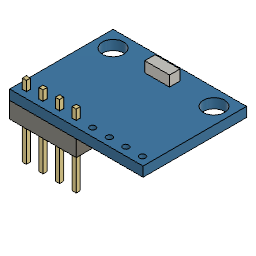
Case_Gyro_Sensor (Autodesk Fusion 360 archive; units mm, degrees)
design "GY-521_MPU6050"
description: Open CASCADE Model
Autodesk Fusion 360 part; units mm, degrees
sketch "Sketch1" plane through (0, 0, 0) normal (0, 0, 1) x (1, 0, 0)
  line L0 (-9.21, -6.355) -> (-8.57, -6.355)
  line L1 (-8.57, -6.355) -> (-8.57, -6.995)
  line L2 (-8.57, -6.995) -> (-9.21, -6.995)
  line L3 (-9.21, -6.995) -> (-9.21, -6.355)
  circle A0 centre (-7.725, 5.425) radius 1.625
  circle A1 centre (7.725, 5.425) radius 1.625
  line L4 (-10.225, 7.925) -> (10.225, 7.925)
  line L5 (10.225, 7.925) -> (10.225, -7.925)
  line L6 (10.225, -7.925) -> (-10.225, -7.925)
  line L7 (-10.225, -7.925) -> (-10.225, 7.925)
  line L8 (-6.03, -6.995) -> (-6.67, -6.995)
  line L9 (-6.67, -6.995) -> (-6.67, -6.355)
  line L10 (-6.67, -6.355) -> (-6.03, -6.355)
  line L11 (-6.03, -6.355) -> (-6.03, -6.995)
  line L12 (-3.49, -6.995) -> (-4.13, -6.995)
  line L13 (-4.13, -6.995) -> (-4.13, -6.355)
  line L14 (-4.13, -6.355) -> (-3.49, -6.355)
  line L15 (-3.49, -6.355) -> (-3.49, -6.995)
  line L16 (-0.95, -6.995) -> (-1.59, -6.995)
  line L17 (-1.59, -6.995) -> (-1.59, -6.355)
  line L18 (-1.59, -6.355) -> (-0.95, -6.355)
  line L19 (-0.95, -6.355) -> (-0.95, -6.995)
  line L20 (1.59, -6.995) -> (0.95, -6.995) construction
  line L21 (0.95, -6.995) -> (0.95, -6.355) construction
  line L22 (0.95, -6.355) -> (1.59, -6.355) construction
  line L23 (1.59, -6.355) -> (1.59, -6.995) construction
  line L24 (4.13, -6.995) -> (3.49, -6.995) construction
  line L25 (3.49, -6.995) -> (3.49, -6.355) construction
  line L26 (3.49, -6.355) -> (4.13, -6.355) construction
  line L27 (4.13, -6.355) -> (4.13, -6.995) construction
  line L28 (6.67, -6.995) -> (6.03, -6.995) construction
  line L29 (6.03, -6.995) -> (6.03, -6.355) construction
  line L30 (6.03, -6.355) -> (6.67, -6.355) construction
  line L31 (6.67, -6.355) -> (6.67, -6.995) construction
  line L32 (9.21, -6.995) -> (8.57, -6.995) construction
  line L33 (8.57, -6.995) -> (8.57, -6.355) construction
  line L34 (8.57, -6.355) -> (9.21, -6.355) construction
  line L35 (9.21, -6.355) -> (9.21, -6.995) construction
  line L36 (-0.95, -6.675) -> (0.95, -6.675) construction
  line L37 (-10.225, -5.425) -> (10.225, -5.425)
  line L38 (10.225, -5.425) -> (10.225, -7.925)
  line L39 (10.225, -7.925) -> (-10.225, -7.925)
  line L40 (-10.225, -7.925) -> (-10.225, -5.425)
  line L41 (0, -5.425) -> (0, -7.925)
  circle A2 centre (1.27, -6.675) radius 0.4525
  circle A3 centre (3.81, -6.675) radius 0.4525
  circle A4 centre (6.35, -6.675) radius 0.4525
  circle A5 centre (8.89, -6.675) radius 0.4525
  line L42 (-2.025, 6.175) -> (1.775, 6.175)
  line L43 (1.775, 6.175) -> (1.775, 4.575)
  line L44 (1.775, 4.575) -> (-2.025, 4.575)
  line L45 (-2.025, 4.575) -> (-2.025, 6.175)
  point P0 (0, -6.675)
  point P1 (0, -5.425)
  point P2 (10.225, 0)
  point P3 (9.21, -6.675)
  point P4 (10.225, -6.675)
  dimension "d1" = 0.64
  dimension "d4" = 2.54
  dimension "d5" = 0
  dimension "d7" = 2.5
  dimension "d8" = 3.25
  dimension "d9" = 2.5
  dimension "d10" = 2.5
  dimension "d11" = 2.5
  dimension "d12" = 15.85
  dimension "d21" = 12
  dimension "d22" = 12.25
  dimension "d23" = 1.6
  dimension "d24" = 1.75
  dimension "d27" = 20.45
  constraint horizontal L0
  constraint vertical L1
  constraint horizontal L2
  constraint vertical L3
  constraint equal L0 L1
  constraint horizontal L4
  constraint vertical L5
  constraint horizontal L6
  constraint vertical L7
  constraint equal A0 A1
  constraint horizontal A0.centre A1.centre
  constraint midpoint L19 L36.start
  constraint midpoint L21 L36.end
  constraint midpoint L36 P0
  constraint vertical origin P0
  constraint horizontal L37
  constraint vertical L38
  constraint horizontal L39
  constraint vertical L40
  constraint coincident L37 P1
  constraint midpoint L37 P1
  constraint vertical P0 P1
  constraint collinear L6 L39
  constraint collinear L5 L38
  constraint collinear L7 L40
  constraint coincident P1 L41.start
  constraint midpoint L6 L41.end
  constraint midpoint L5 P2
  constraint horizontal origin P2
  constraint midpoint L35 P3
  constraint midpoint L38 P4
  constraint horizontal P3 P4
  constraint coincident L21.end A2
  constraint coincident L22.end A2
  constraint coincident L20.start A2
  constraint coincident L25.end A3
  constraint coincident L26.end A3
  constraint coincident L24.start A3
  constraint coincident L29.end A4
  constraint coincident L30.end A4
  constraint coincident L28.start A4
  constraint coincident L32.end A5
  constraint coincident L33.end A5
  constraint coincident L32.start A5
  constraint horizontal L42
  constraint vertical L43
  constraint horizontal L44
  constraint vertical L45
  measures "d1" distance of L0.start L0.end
  measures "d7" distance of L37.end L5.end
  measures "d8" diameter of A0
  measures "d9" distance of A0.centre L7
  measures "d10" distance of A1.centre L5
  measures "d11" distance of A0.centre L4
  measures "d12" distance of L4.end L5.end
  measures "d21" distance of L7 L43
  measures "d22" distance of L5 L45
  measures "d23" distance of L42 L44
  measures "d24" distance of L4 L42
  measures "d27" distance of L5.end L6.end
extrude "Extrude1" add sketch "Sketch1" against normal blind 1.5 contours L4 L5 L7 L37 | L6 L7 L37 L39 L40 L41 | L5 L6 L37 L38 L39 L41 | L42 L43 L44 L45 makes body 1
extrude "Extrude2" add sketch "Sketch1" against normal blind 11.15 from surface at 1.5 separate body contours L0 L1 L2 L3 | L8 L9 L10 L11 | L12 L13 L14 L15 | L16 L17 L18 L19 makes body 2 at (-6.2433, -6.995, -5.9333) makes body 3 at (-3.7033, -6.995, -2.2167) makes body 4 at (-8.9967, -6.355, -5.9333) makes body 5 at (-1.1633, -6.995, -5.9333)
extrude "Extrude3" add sketch "Sketch1" against normal blind 2.5 from surface at -1.5 separate body contours L6 L7 L37 L39 L40 L41 makes body 6
extrude "Extrude4" add sketch "Sketch1" along normal blind 1.6 separate body contours L42 L43 L44 L45 makes body 7
equation "d9 = d11"
equation "d10 = d9"
